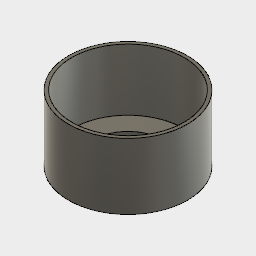
Case_Cap (Autodesk Fusion 360 design; units mm, degrees)
Autodesk Fusion 360 part; units mm, degrees
sketch "Sketch1" plane through (0, 0, 0) normal (0, 1, 0) x (1, 0, 0)
  circle A0 centre (0, 0) radius 13.5
  circle A1 centre (0, 0) radius 8.25
  dimension "d1" = 27
  dimension "d7" = 16.5
  measures "d1" diameter of A0
  measures "d7" diameter of A1
extrude "Extrude1" add sketch "Sketch1" along normal blind 15
sketch "Sketch2" plane through (0, 15, 0) normal (0, 1, 0) x (-1, 0, 0)
  circle A0 centre (0, 0) radius 13.5
  circle A1 centre (0, 0) radius 12.75
  circle A2 centre (0, 0) radius 8.25
  dimension "d4" = 25.5
  measures "d4" diameter of A1
extrude "Extrude2" cut sketch "Sketch2" against normal blind 14 contours A1 | A2
